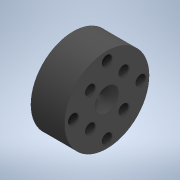
# Autodesk Inventor part: baseSoporte
Saved by Autodesk Inventor 2021.5 (Build 255421000, 421)
## iProperties
Created: 2024-11-19
Part Number: baseSoporte
Material: ABS NEGRO 4DLAB
Document SubType Name: Modeling
Designer: Joho_
Density: 0.894 g/cm^3
Appearance: Genérico(2)
Mass: 23.9494 g
Surface Area: 100.952 cm^2
Volume: 26.789 cm^3
Author: Joho_
## iProperties of the stored document _3DPrint.ipt
Created: 2024-11-25
Part Number: _3DPrint
Material: Genérico
Document SubType Name: Modeling
Designer: Joho_
Density: 1 g/cm^3
Appearance: Valor por defecto
Author: Joho_
Autodesk Inventor part; units mm, degrees
ref_plane "YZ Plane" through (0, 0, 0) normal (1, 0, 0) x (0, 1, 0)
sketch "Boceto2" plane through (0, 0, 0) normal (0, 0, 1) x (1, 0, 0)
  line L0 (0, 0) -> (-71.5, 0)
  line L1 (0, 10.9) -> (0, 0)
  line L2 (-68.2708, 0) -> (0, 0)
  line L3 (0, 10.9) -> (-68.1013, 9.2541)
  line L4 (-71.5, 0) -> (-56.9274, 0) construction
  line L5 (-71.5, 0) -> (-71.5, 8.5)
  line L6 (-71.5, 0) -> (-68, 0)
  arc A0 (-68, 9.2565) -> (-71.5, 8.5) centre (-67.8264, -0.0207) ccw
  line L7 (-68, 9.2565) -> (0, 10.9)
  line L8 (0, 0) -> (26.5, 0)
  line L9 (26.5, 0) -> (26.5, 7)
  line L10 (0, 0) -> (0, 9.9)
  line L11 (0, 0) -> (21, 0)
  line L12 (21, 0) -> (21, 9.5)
  line L13 (21, 9.5) -> (0, 9.9)
  line L14 (26.5, 0) -> (26.5, 8.5)
  arc A1 (26.5, 8.5) -> (21, 9.5) centre (21.692, -2.3188) ccw
  line L15 (26.5, 0) -> (29, 0)
  line L16 (29, 0) -> (29, 7)
  line L17 (29, 7) -> (26.5, 7)
  line L18 (29, 0) -> (29, 6.75)
  line L19 (29, 6.75) -> (31, 6.75)
  line L20 (31.8816, 0) -> (29, 0)
  line L21 (29, 0) -> (29, 6.75)
  line L22 (29, 6.75) -> (31, 6.75)
  line L23 (29, 0) -> (31, 0)
  ellipse E0 centre (31, 0) end of major axis (31, 6.75) minor radius 0.8816 (31.8816, 0) -> (31, 6.75) ccw
  line L24 (-71.5, 0) -> (-71.5, 7.25)
  line L25 (-71.5, 0) -> (-67, 0)
  line L26 (-71.5, 0) -> (-76, 0)
  line L27 (-76, 0) -> (-76, 6.75)
  line L28 (-76, 6.75) -> (-71.5, 7.25)
  line L29 (-76, 0) -> (-77, 0)
  line L30 (-77, 0) -> (-77, 6.5)
  line L31 (-77, 6.5) -> (-76, 6.75)
  line L32 (-77, 0) -> (-80.5, 0)
  line L33 (-80.5, 0) -> (-80.5, 4.15)
  line L34 (-80.5, 4.15) -> (-77, 6.5)
  line L35 (-80.5, 0) -> (-87.5, 0)
  line L36 (-87.5, 0) -> (-87.5, 4.15)
  line L37 (-87.5, 4.15) -> (-80.5, 4.15)
  line L38 (-80.5, 4.15) -> (-80.5, 0)
  line L39 (-87.5, 0) -> (-95, 0)
  line L40 (-95, 0) -> (-95, 0)
  line L41 (-92.25, 2.75) -> (-87.5, 2.75)
  line L42 (-87.5, 2.75) -> (-87.5, 0)
  arc A2 (-92.25, 2.75) -> (-95, 0) centre (-92.25, 0) ccw
  line L43 (-71.5, 8.5) -> (-71.5, 12.7399)
  arc A3 (-68.0867, 13.2556) -> (-71.5, 12.7399) centre (-67.8264, -0.0207) ccw
  line L44 (-68.0867, 13.2556) -> (-0.0966, 14.8988)
  line L45 (34.8792, 10.8985) -> (49.8792, 10.8985)
  line L46 (-71.5, 0) -> (-61.5, 0)
  line L47 (-61.5, 0) -> (-61.5, 13.4148)
  line L48 (-61.5, 14.4151) -> (-61.5, 20)
  line L49 (-61.5, 13.4148) -> (-61.5, 14.4151)
  line L50 (-61.5, 13.4148) -> (-58, 13.4148) construction
  circle A4 centre (-61.5, 13.4148) radius 1.5
  line L51 (-61.5, 13.4148) -> (-58.5, 13.4148)
  line L52 (-58.5, 13.4148) -> (-60, 10.8167)
  line L53 (-60, 10.8167) -> (-63, 10.8167)
  line L54 (-63, 10.8167) -> (-64.5, 13.4148)
  line L55 (-64.5, 13.4148) -> (-63, 16.0129)
  line L56 (-63, 16.0129) -> (-60, 16.0129)
  line L57 (-60, 16.0129) -> (-58.5, 13.4148)
  line L58 (-64.7321, 19.0129) -> (-67.9641, 13.4148)
  line L59 (-67.9641, 13.4148) -> (-64.7321, 7.8167)
  line L60 (-64.7321, 7.8167) -> (-58.2679, 7.8167)
  line L61 (-58.2679, 7.8167) -> (-55.0359, 13.4148)
  line L62 (-55.0359, 13.4148) -> (-58.2679, 19.0129)
  line L63 (-58.2679, 19.0129) -> (-64.7321, 19.0129)
  line L64 (-67.9641, 13.4148) -> (-55.0359, 13.4148)
  line L65 (49.8792, 0) -> (39.8792, 0)
  line L66 (-71.5, 0) -> (-10.8105, 0)
  line L67 (-10.8105, 0) -> (-10.8105, 14.6399)
  line L68 (-10.8105, 14.6399) -> (-10.8105, 27)
  circle A5 centre (-10.8105, 14.6399) radius 1.5
  line L69 (-10.8105, 14.6399) -> (-7.8105, 14.6399)
  line L70 (-10.8105, 14.6399) -> (-7.8105, 14.6399) construction
  line L71 (-7.8105, 14.6399) -> (-9.3105, 12.0418)
  line L72 (-9.3105, 12.0418) -> (-12.3105, 12.0418)
  line L73 (-12.3105, 12.0418) -> (-13.8105, 14.6399)
  line L74 (-13.8105, 14.6399) -> (-12.3105, 17.238)
  line L75 (-12.3105, 17.238) -> (-9.3105, 17.238)
  line L76 (-9.3105, 17.238) -> (-7.8105, 14.6399)
  line L77 (-14.0426, 20.238) -> (-17.2746, 14.6399)
  line L78 (-17.2746, 14.6399) -> (-14.0426, 9.0418)
  line L79 (-14.0426, 9.0418) -> (-7.5784, 9.0418)
  line L80 (-7.5784, 9.0418) -> (-4.3464, 14.6399)
  line L81 (-4.3464, 14.6399) -> (-7.5784, 20.238)
  line L82 (-7.5784, 20.238) -> (-14.0426, 20.238)
  line L83 (0, 10.9) -> (50, 10.9)
  line L84 (50, 10.9) -> (50, 14.9)
  line L85 (50, 14.9) -> (0, 14.9)
  line L86 (0, 14.9) -> (0, 10.9)
  line L87 (-0.0966, 14.8988) -> (0, 14.8988)
  line L88 (0, 0) -> (50, 0)
  line L89 (50, 0) -> (50, 10.9)
  line L90 (50, 10.9) -> (0, 10.9)
  line L91 (0, 10.9) -> (0, 0)
  point P0 (67.7333, -10.8479)
  point P1 (103.6012, -10.8479)
  point P2 (35.8517, 0)
  point P3 (7, 16)
  point P4 (-95, 2.75)
  dimension "d21" = 71.5
  dimension "d22" = 8.5
  dimension "d23" = 3.5
  dimension "d24" = 26.5
  dimension "d25" = 7
  dimension "d26" = 9.9
  dimension "d27" = 21
  dimension "d28" = 9.5
  dimension "d29" = 8.5
  dimension "d30" = 2.5
  dimension "d31" = 6.75
  dimension "d32" = 2
  dimension "d33" = 2
  dimension "d34" = 7.25
  dimension "d35" = 4.5
  dimension "d36" = 4.5
  dimension "d37" = 6.75
  dimension "d38" = 1
  dimension "d39" = 6.5
  dimension "d40" = 3.5
  dimension "d41" = 4.15
  dimension "d42" = 7
  dimension "d43" = 7.5
  dimension "d44" = 2.75
  dimension "d45" = 2.75
  dimension "d51" = 4
  dimension "d52" = 10
  dimension "d53" = 20
  dimension "d54" = 90
  dimension "d55" = 3
  dimension "d56" = 3
  dimension "d57" = 3
  dimension "d58" = 10
  dimension "d63" = 60.6895
  dimension "d64" = 3
  dimension "d65" = 3
  dimension "d66" = 0
  dimension "d67" = 3
  dimension "d89" = 50
  dimension "d90" = 4
  dimension "d91" = 121.5
  dimension "d92" = 50
  constraints: 184 end point, 19 horizontal, 17 point on line, 12 perpendicular, 10 coincident, 9 parallel, 9 point on circle, 6 centre point, 6 vertical, 2 collinear, 2 tangent, 40 other
  measures "d21" distance of L0.start L0.end
  measures "d22" distance of L0.end L5.end
  measures "d23" distance of L0.end L6.end
  measures "d24" distance of L0.start L8.end
  measures "d25" distance of L8.end L9.end
  measures "d26" distance of L0.start L10.end
  measures "d27" distance of L0.start L11.end
  measures "d28" distance of L11.end L12.end
  measures "d29" distance of L8.end L14.end
  measures "d30" distance of L8.end L15.end
  measures "d31" distance of L15.end L18.end
  measures "d32" distance of L18.end L19.end
  measures "d33" distance of L20.end L23.end
  measures "d34" distance of L0.end L24.end
  measures "d35" distance of L0.end L25.end
  measures "d36" distance of L0.end L26.end
  measures "d37" distance of L26.end L27.end
  measures "d38" distance of L26.end L29.end
  measures "d39" distance of L29.end L30.end
  measures "d40" distance of L29.end L32.end
  measures "d41" distance of L32.end L33.end
  measures "d42" distance of L36.end L37.end
  measures "d43" distance of point (-95, 2.75) L41.end
  measures "d44" distance of L39.end point (-95, 2.75)
  measures "d45" radius of A2
  measures "d51" radial gap between concentric circles of A0 A3
  measures "d52" distance of L0.end L46.end
  measures "d53" distance of L46.end L48.end
  measures "d54" angle of L47 L46
  measures "d55" diameter of A4
  measures "d56" distance of L51.start L51.end
  measures "d57" distance between parallel lines of L55 L58
  measures "d58" distance of L65.start L65.end
  measures "d63" distance of L0.end L66.end
  measures "d64" diameter of A5
  measures "d65" distance of L69.start L69.end
  measures "d66" distance between parallel lines of L69 L70
  measures "d67" distance between parallel lines of L74 L77
  measures "d89" distance of L85.end L84.end
  measures "d90" distance of L84.end L83.end
  measures "d91" distance between parallel lines of L84 L24
  measures "d92" distance between parallel lines of L86 L84
sketch "Boceto4" plane through (0, 0, 0) normal (1, 0, 0) x (0, 1, 0)
  line L0 (0, 0) -> (0, 20)
  circle A0 centre (20, 0) radius 3
  circle A1 centre (0, 20) radius 3
  circle A2 centre (-20, 0) radius 3
  circle A3 centre (0, 0) radius 12.5
  circle A4 centre (0, 0) radius 20
  circle A5 centre (0, 0) radius 20
  circle A6 centre (0, 0) radius 20
  circle A7 centre (0, 0) radius 25
  circle A8 centre (0, 0) radius 20
  circle A9 centre (0, -20) radius 3
  line L1 (0, -20) -> (3.5355, -16.4645) construction
  circle A10 centre (9.9038, -9.9038) radius 1.5
  line L2 (0, 0) -> (6.2936, 0)
  line L3 (15, 15) -> (-15, 15)
  line L4 (-15, 15) -> (-15, -15)
  line L5 (-15, -15) -> (15, -15)
  line L6 (15, -15) -> (15, 15)
  line L7 (15, 15) -> (-15, -15) construction
  line L8 (8.3161, -12.6538) -> (6.7284, -9.9038)
  line L9 (6.7284, -9.9038) -> (8.3161, -7.1538)
  line L10 (8.3161, -7.1538) -> (11.4915, -7.1538)
  line L11 (11.4915, -7.1538) -> (13.0792, -9.9038)
  line L12 (13.0792, -9.9038) -> (11.4915, -12.6538)
  line L13 (11.4915, -12.6538) -> (8.3161, -12.6538)
  circle A11 centre (9.9038, 9.9038) radius 1.5
  line L14 (8.3161, 12.6538) -> (6.7284, 9.9038)
  line L15 (6.7284, 9.9038) -> (8.3161, 7.1538)
  line L16 (8.3161, 7.1538) -> (11.4915, 7.1538)
  line L17 (11.4915, 7.1538) -> (13.0792, 9.9038)
  line L18 (13.0792, 9.9038) -> (11.4915, 12.6538)
  line L19 (11.4915, 12.6538) -> (8.3161, 12.6538)
  circle A12 centre (-9.9038, -9.9038) radius 1.5
  line L20 (-8.3161, -12.6538) -> (-6.7284, -9.9038)
  line L21 (-6.7284, -9.9038) -> (-8.3161, -7.1538)
  line L22 (-8.3161, -7.1538) -> (-11.4915, -7.1538)
  line L23 (-11.4915, -7.1538) -> (-13.0792, -9.9038)
  line L24 (-13.0792, -9.9038) -> (-11.4915, -12.6538)
  line L25 (-11.4915, -12.6538) -> (-8.3161, -12.6538)
  line L26 (-13.0792, 9.9038) -> (-11.4915, 12.6538)
  line L27 (-8.3161, 7.1538) -> (-11.4915, 7.1538)
  line L28 (-6.7284, 9.9038) -> (-8.3161, 7.1538)
  line L29 (-11.4915, 7.1538) -> (-13.0792, 9.9038)
  circle A13 centre (-9.9038, 9.9038) radius 1.5
  line L30 (-8.3161, 12.6538) -> (-6.7284, 9.9038)
  line L31 (-11.4915, 12.6538) -> (-8.3161, 12.6538)
  circle A14 centre (9.9038, 9.9038) radius 3
  circle A15 centre (9.9038, -9.9038) radius 3
  circle A16 centre (-9.9038, 9.9038) radius 3
  circle A17 centre (-9.9038, -9.9038) radius 3
  point P0 (20, 0)
  point P1 (-6.2936, 0)
  dimension "d105" = 40
  dimension "d104" = 50
  dimension "d107" = 6
  dimension "d108" = 360
  dimension "d110" = 25
  dimension "d126" = 3
  dimension "d132" = 30
  dimension "d133" = 30
  dimension "d270" = 6
  dimension "d271" = 6
  dimension "d272" = 6
  dimension "d273" = 6
  constraints: 64 end point, 25 symmetric about line, 14 centre point, 12 coincident, 2 horizontal, 2 horizontal alignment, 2 parallel, 2 vertical alignment, 1 midpoint, 1 perpendicular, 43 other
  measures "d104" diameter of A7
  measures "d107" diameter of A1
  measures "d110" diameter of A3
  measures "d126" diameter of A10
  measures "d132" distance of L5.end L4.end
  measures "d133" distance of L4.end L3.end
  measures "d270" diameter of A14
  measures "d271" diameter of A15
  measures "d272" diameter of A16
  measures "d273" diameter of A17
sketch "Boceto3" plane through (0, 0, 0) normal (1, 0, 0) x (0, 1, 0)
  line L0 (0, 0) -> (20, 0) construction
  line L1 (0, 0) -> (14.1421, 14.1421)
  circle A0 centre (0, 20) radius 3
  circle A1 centre (14.1421, -14.1421) radius 3
  circle A2 centre (14.1421, 14.1421) radius 3
  circle A3 centre (-14.1421, 14.1421) radius 3
  circle A4 centre (0, 0) radius 12.5
  circle A5 centre (0, 0) radius 20
  circle A6 centre (0, 0) radius 20
  circle A7 centre (0, 0) radius 20
  circle A8 centre (0, 0) radius 25
  circle A9 centre (0, 0) radius 20
  circle A10 centre (-14.1421, -14.1421) radius 3
  line L2 (20, 0) -> (20, 4)
  line L3 (20, 4) -> (23.4641, 2)
  line L4 (23.4641, 2) -> (23.4641, -2)
  line L5 (23.4641, -2) -> (20, -4)
  line L6 (20, -4) -> (16.5359, -2)
  line L7 (16.5359, -2) -> (16.5359, 2)
  line L8 (16.5359, 2) -> (20, 4)
  line L9 (-4, 20) -> (-2, 23.4641)
  line L10 (-2, 23.4641) -> (2, 23.4641)
  line L11 (2, 23.4641) -> (4, 20)
  line L12 (4, 20) -> (2, 16.5359)
  line L13 (-2, 16.5359) -> (-4, 20)
  line L14 (2, 16.5359) -> (-2, 16.5359)
  line L15 (-20, -4) -> (-23.4641, -2)
  line L16 (-23.4641, -2) -> (-23.4641, 2)
  line L17 (-23.4641, 2) -> (-20, 4)
  line L18 (-20, 4) -> (-16.5359, 2)
  line L19 (-16.5359, -2) -> (-20, -4)
  line L20 (-16.5359, 2) -> (-16.5359, -2)
  line L21 (4, -20) -> (2, -23.4641)
  line L22 (2, -23.4641) -> (-2, -23.4641)
  line L23 (-2, -23.4641) -> (-4, -20)
  line L24 (-4, -20) -> (-2, -16.5359)
  line L25 (2, -16.5359) -> (4, -20)
  line L26 (-2, -16.5359) -> (2, -16.5359)
  circle A11 centre (20, 0) radius 2
  circle A12 centre (0, 20) radius 2
  circle A13 centre (-20, 0) radius 2
  circle A14 centre (0, -20) radius 2
  line L27 (-14.1421, -14.1421) -> (-17.6777, -17.6777)
  line L28 (-14.1421, -14.1421) -> (-9.1421, -14.1421) construction
  line L29 (-17.6777, -17.6777) -> (17.6777, -17.6777)
  line L30 (17.6777, -17.6777) -> (17.6777, 17.6777)
  line L31 (17.6777, -17.6777) -> (59.3553, -17.6777) construction
  line L32 (17.6777, 17.6777) -> (-17.6777, 17.6777)
  line L33 (17.6777, 17.6777) -> (68.3553, 17.6777) construction
  line L34 (-17.6777, 17.6777) -> (-17.6777, -17.6777)
  dimension "d75" = 40
  dimension "d74" = 50
  dimension "d76" = 45
  dimension "d77" = 6
  dimension "d78" = 360
  dimension "d79" = 6
  dimension "d80" = 25
  dimension "d81" = 4
  dimension "d82" = 360
  dimension "d83" = 4
  dimension "d84" = 360
  dimension "d85" = 135
  dimension "d86" = 45
  dimension "d87" = 90
  dimension "d88" = 180
  constraints: 70 end point, 12 centre point, 11 coincident, 6 point on circle, 4 horizontal, 2 coincident with centre, 2 equal length, 2 vertical, 97 other
  measures "d74" diameter of A8
  measures "d76" angle of L0 L1
  measures "d77" diameter of A2
  measures "d79" diameter of A0
  measures "d80" diameter of A4
  measures "d81" distance of L0.end L2.end
  measures "d83" diameter of A11
  measures "d85" angle of L27 L28
  measures "d86" angle of L29 L27
  measures "d87" angle of L31 L30
  measures "d88" angle of L32 L33
extrude "Extrusión2" add sketch "Boceto4" along normal blind 50 and the other way blind 71.5 contours L3 A4 L6 L5 L4 | A3 A14 L14 L15 L16 A15 L10 L9 L8 A17 L20 L21 L22 A16 L27 L28 L30 | A14 L14 A3 | A3 L14 A14 | A16 L30 A3 | A3 L30 A16 | L3 L6 A4 | A4 L4 L3 | L14 A14 L19 L18 L17 L16 A3 | A3 L16 A14 L15 L14 | L14 L19 A14 | A14 L15 L14 | L30 A16 L28 L27 A3 | A3 L27 A16 L29 L26 L31 L30 | L30 L28 A16 | A16 L31 L30 | L16 A14 A3 | A3 A14 L16 | A14 L19 | L15 A14 | L27 A16 A3 | A3 A16 L27 | L31 A16 | L6 L5 A4 | A4 L5 L4 | L16 L15 A14 | A14 L17 L16 | L19 L18 A14 | A16 L28 L27 | L27 L29 A16 | A16 L28 | A16 L26 L31 | L17 A14 | A14 L18 | A17 L22 A3 | A3 L22 A17 | A16 L29 | L26 A16 | A15 L10 A3 | A3 L10 A15 | A14 L18 L17 | L22 A17 L21 L20 A3 | A3 L20 A17 L25 L24 L23 L22 | L22 L21 A17 | A17 L23 L22 | L29 L26 A16 | L10 A15 L11 L12 L13 L8 A3 | A3 L8 A15 L9 L10 | L10 L11 A15 | A15 L9 L10 | L20 A17 A3 | A3 A17 L20 | A17 L21 | L23 A17 | L8 A15 A3 | A3 A15 L8 | A15 L11 | L9 A15 | L20 L25 A17 | A17 L21 L20 | A17 L24 L23 | A15 L13 L8 | L8 L9 A15 | L11 L12 A15 | A17 L25 | L24 A17 | L13 A15 | L25 L24 A17 | A15 L12 L13 | A15 L12 | A10 | A11 | A12 | A13
revolve "Revolución2" cut sketch "Boceto2" angle 360 about axis through (-71.5, 0, 0) along (1, 0, 0) contours L0 L67 L79 L80 L3 L1 | L1 L13 L12 L8 | L0 L47 L60 L61 L3 L78 L79 L67 | L1 L83 L45 L89 L88 L65 E0 L19 L16 L17 L14 A1 L13 | L12 A1 L14 L9 L8 | L0 L5 A0 L3 L59 L60 L47 | L79 L78 L3 L67 | L67 L3 L80 L79 | L9 L17 L16 L15 | L60 L59 L3 L47 | L47 L3 L61 L60 | L16 L19 E0 L20
sketch "Boceto5" plane through (50, 0, 0) normal (1, 0, 0) x (0, 0, -1)
  line L0 (0, 0) -> (0, 20)
  circle A0 centre (20, 0) radius 3
  circle A1 centre (0, 20) radius 3
  circle A2 centre (-20, 0) radius 3
  circle A3 centre (0, 0) radius 20
  circle A4 centre (0, 0) radius 20
  circle A5 centre (0, 0) radius 20
  circle A6 centre (0, 0) radius 20
  circle A7 centre (0, -20) radius 3
  line L1 (0, -20) -> (3.5355, -16.4645) construction
  circle A8 centre (9.9038, -9.9038) radius 1.5
  line L2 (0, 0) -> (6.2936, 0)
  line L3 (15, 15) -> (-15, 15)
  line L4 (-15, 15) -> (-15, -15)
  line L5 (-15, -15) -> (15, -15)
  line L6 (15, -15) -> (15, 15)
  line L7 (15, 15) -> (-15, -15) construction
  line L8 (8.3161, -12.6538) -> (6.7284, -9.9038)
  line L9 (6.7284, -9.9038) -> (8.3161, -7.1538)
  line L10 (8.3161, -7.1538) -> (11.4915, -7.1538)
  line L11 (11.4915, -7.1538) -> (13.0792, -9.9038)
  line L12 (13.0792, -9.9038) -> (11.4915, -12.6538)
  line L13 (11.4915, -12.6538) -> (8.3161, -12.6538)
  line L14 (13.0792, 9.9038) -> (11.4915, 12.6538)
  line L15 (8.3161, 7.1538) -> (11.4915, 7.1538)
  line L16 (6.7284, 9.9038) -> (8.3161, 7.1538)
  line L17 (11.4915, 7.1538) -> (13.0792, 9.9038)
  circle A9 centre (9.9038, 9.9038) radius 1.5
  line L18 (8.3161, 12.6538) -> (6.7284, 9.9038)
  line L19 (11.4915, 12.6538) -> (8.3161, 12.6538)
  line L20 (-8.3161, -7.1538) -> (-11.4915, -7.1538)
  line L21 (-13.0792, -9.9038) -> (-11.4915, -12.6538)
  line L22 (-8.3161, -12.6538) -> (-6.7284, -9.9038)
  circle A10 centre (-9.9038, -9.9038) radius 1.5
  line L23 (-6.7284, -9.9038) -> (-8.3161, -7.1538)
  line L24 (-6.7284, 9.9038) -> (-8.3161, 7.1538)
  line L25 (-8.3161, 7.1538) -> (-11.4915, 7.1538)
  line L26 (-11.4915, 7.1538) -> (-13.0792, 9.9038)
  line L27 (-13.0792, 9.9038) -> (-11.4915, 12.6538)
  line L28 (-8.3161, 12.6538) -> (-6.7284, 9.9038)
  line L29 (-11.4915, 12.6538) -> (-8.3161, 12.6538)
  line L30 (-11.4915, -7.1538) -> (-13.0792, -9.9038)
  circle A11 centre (-9.9038, 9.9038) radius 1.5
  line L31 (-11.4915, -12.6538) -> (-8.3161, -12.6538)
  circle A12 centre (0, 0) radius 25
  point P0 (20, 0)
  point P1 (-6.2936, 0)
  dimension "d144" = 40
  dimension "d145" = 6
  dimension "d146" = 360
  dimension "d148" = 3
  dimension "d149" = 30
  dimension "d150" = 30
  dimension "d182" = 50
  constraints: 64 end point, 25 symmetric about line, 9 centre point, 7 coincident, 2 horizontal, 2 horizontal alignment, 2 parallel, 2 vertical alignment, 1 midpoint, 1 perpendicular, 43 other
  measures "d145" diameter of A1
  measures "d148" diameter of A8
  measures "d149" distance of L5.end L4.end
  measures "d150" distance of L4.end L3.end
  measures "d182" diameter of A12
extrude "Extrusión3" cut sketch "Boceto5" against normal blind 20 contours A8 | A9 | A10 | A11
ref_plane "Plano de trabajo1" through (45, 0, 0) normal (1, 0, 0) x (0, 0, -1)
sketch "Boceto8" plane through (45, 0, 0) normal (1, 0, 0) x (0, 0, -1)
  line L0 (0, 0) -> (0, 20)
  circle A0 centre (20, 0) radius 3
  circle A1 centre (0, 20) radius 3
  circle A2 centre (-20, 0) radius 3
  circle A3 centre (0, 0) radius 20
  circle A4 centre (0, 0) radius 20
  circle A5 centre (0, 0) radius 20
  circle A6 centre (0, 0) radius 20
  circle A7 centre (0, -20) radius 3
  line L1 (0, -20) -> (3.5355, -16.4645) construction
  circle A8 centre (9.9038, -9.9038) radius 1.5
  line L2 (0, 0) -> (6.2936, 0)
  line L3 (15, 15) -> (-15, 15)
  line L4 (-15, 15) -> (-15, -15)
  line L5 (-15, -15) -> (15, -15)
  line L6 (15, -15) -> (15, 15)
  line L7 (8.3161, -12.6538) -> (6.7284, -9.9038)
  line L8 (6.7284, -9.9038) -> (8.3161, -7.1538)
  line L9 (8.3161, -7.1538) -> (11.4915, -7.1538)
  line L10 (11.4915, -7.1538) -> (13.0792, -9.9038)
  line L11 (13.0792, -9.9038) -> (11.4915, -12.6538)
  line L12 (11.4915, -12.6538) -> (8.3161, -12.6538)
  line L13 (13.0792, 9.9038) -> (11.4915, 12.6538)
  line L14 (8.3161, 7.1538) -> (11.4915, 7.1538)
  line L15 (6.7284, 9.9038) -> (8.3161, 7.1538)
  line L16 (11.4915, 7.1538) -> (13.0792, 9.9038)
  circle A9 centre (9.9038, 9.9038) radius 1.5
  line L17 (8.3161, 12.6538) -> (6.7284, 9.9038)
  line L18 (11.4915, 12.6538) -> (8.3161, 12.6538)
  line L19 (-8.3161, -7.1538) -> (-11.4915, -7.1538)
  line L20 (-13.0792, -9.9038) -> (-11.4915, -12.6538)
  line L21 (-8.3161, -12.6538) -> (-6.7284, -9.9038)
  circle A10 centre (-9.9038, -9.9038) radius 1.5
  line L22 (-6.7284, -9.9038) -> (-8.3161, -7.1538)
  line L23 (-6.7284, 9.9038) -> (-8.3161, 7.1538)
  line L24 (-8.3161, 7.1538) -> (-11.4915, 7.1538)
  line L25 (-11.4915, 7.1538) -> (-13.0792, 9.9038)
  line L26 (-13.0792, 9.9038) -> (-11.4915, 12.6538)
  line L27 (-8.3161, 12.6538) -> (-6.7284, 9.9038)
  line L28 (-11.4915, 12.6538) -> (-8.3161, 12.6538)
  line L29 (-11.4915, -7.1538) -> (-13.0792, -9.9038)
  circle A11 centre (-9.9038, 9.9038) radius 1.5
  line L30 (-11.4915, -12.6538) -> (-8.3161, -12.6538)
  line L31 (15, -15) -> (15, 15)
  line L32 (11.4915, -12.6538) -> (15, -12.6538)
  line L33 (15, -12.6538) -> (15, -7.1538)
  line L34 (15, -7.1538) -> (11.4915, -7.1538)
  line L35 (11.4915, -7.1538) -> (11.4915, -12.6538)
  line L36 (11.4915, 7.1538) -> (15, 7.1538)
  line L37 (15, 7.1538) -> (15, 12.6538)
  line L38 (15, 12.6538) -> (11.4915, 12.6538)
  line L39 (11.4915, 12.6538) -> (11.4915, 7.1538)
  line L40 (-11.4915, 12.6538) -> (-17.8424, 12.6538)
  line L41 (-17.8424, 12.6538) -> (-17.8424, 7.1538)
  line L42 (-17.8424, 7.1538) -> (-11.4915, 7.1538)
  line L43 (-11.4915, 7.1538) -> (-11.4915, 12.6538)
  line L44 (-11.4915, -7.1538) -> (-17.8424, -7.1538)
  line L45 (-17.8424, -7.1538) -> (-17.8424, -12.6538)
  line L46 (-17.8424, -12.6538) -> (-11.4915, -12.6538)
  line L47 (-11.4915, -12.6538) -> (-11.4915, -7.1538)
  point P0 (20, 0)
  point P1 (-6.2936, 0)
  dimension "d172" = 40
  dimension "d173" = 6
  dimension "d174" = 360
  dimension "d175" = 3
  dimension "d176" = 30
  dimension "d177" = 30
  dimension "d178" = 5.5
  dimension "d179" = 5.5
  constraints: 96 end point, 8 centre point, 6 coincident, 4 parallel, 2 horizontal, 2 horizontal alignment, 2 perpendicular, 2 point on line, 2 vertical alignment, 40 other
  measures "d173" diameter of A1
  measures "d175" diameter of A8
  measures "d176" distance of L6.start L4.end
  measures "d177" distance of L4.end L3.end
  measures "d178" distance of L33.end L32.end
  measures "d179" distance of L37.end L36.end
extrude "Extrusión4" cut sketch "Boceto8" along normal mid plane 2.5 contours L6 L36 L16 L13 L38 | L40 L4 L42 L41 A3 | A3 L41 L40 | L40 L26 L25 L42 L4 | L39 L14 L15 L17 L18 | L13 L16 L39 | L43 L25 L26 | L28 L27 L23 L24 L43 | L6 L32 L11 L10 L34 | L44 L29 L20 L46 L4 | L4 L46 A3 L45 L44 | L35 L12 L7 L8 L9 | L10 L11 L35 | L47 L20 L29 | L19 L22 L21 L30 L47 | A3 L46 L45 | A8 | A9 | A10 | A11
sketch "Boceto9" plane through (50, 0, 0) normal (1, 0, 0) x (0, 0, -1)
  circle A0 centre (20, 0) radius 3
  circle A1 centre (0, 20) radius 3
  circle A2 centre (-20, 0) radius 3
  circle A3 centre (0, 0) radius 12.5
  circle A4 centre (0, 0) radius 20
  circle A5 centre (0, 0) radius 20
  circle A6 centre (0, 0) radius 20
  circle A7 centre (0, 0) radius 25
  circle A8 centre (0, 0) radius 20
  circle A9 centre (0, -20) radius 3
  line L0 (0, -20) -> (3.5355, -16.4645) construction
  line L1 (0, 0) -> (6.2936, 0)
  circle A10 centre (0, 0) radius 2
  circle A11 centre (0, 0) radius 4
  line L2 (-15, 15) -> (15, 15)
  line L3 (15, 15) -> (15, -15)
  line L4 (15, -15) -> (-15, -15)
  line L5 (-15, -15) -> (-15, 15)
  line L6 (-15, 15) -> (15, -15) construction
  line L7 (15, 15) -> (-15, -15) construction
  point P0 (20, 0)
  point P1 (-6.2936, 0)
  point P2 (-15, -13.2288)
  point P3 (-19.775, -2.9916)
  point P4 (-19.775, 2.9916)
  point P5 (-15, 13.2288)
  point P6 (-13.2288, 15)
  point P7 (-2.9916, 19.775)
  point P8 (2.9916, 19.775)
  point P9 (13.2288, 15)
  dimension "d187" = 40
  dimension "d186" = 50
  dimension "d188" = 6
  dimension "d189" = 360
  dimension "d190" = 25
  dimension "d194" = 4
  dimension "d195" = 8
  dimension "d244" = 30
  dimension "d245" = 30
  constraints: 16 end point, 10 coincident, 8 centre point, 2 horizontal, 2 horizontal alignment, 2 midpoint, 2 parallel, 1 perpendicular, 1 vertical alignment, 28 other
  measures "d186" diameter of A7
  measures "d188" diameter of A1
  measures "d190" diameter of A3
  measures "d194" diameter of A10
  measures "d195" diameter of A11
  measures "d244" distance of L3.end L4.end
  measures "d245" distance of L2.end L3.end
extrude "Extrusión5" add sketch "Boceto9" along normal blind 10 contours A0 A4 L3 | L3 A4 L4 L5 L2 | A4 L2 L3 | L3 L4 A4 | L2 A4 A1 | A4 A9 L4 | A4 L5 L2 | L4 L5 A4 | L5 A4 A2 | A3 | A7 | A11
ref_plane "Plano de trabajo2" through (0, 0, 15) normal (0, 0, 1) x (1, 0, 0)
extrude "Extrusión10" add sketch "Boceto9" against normal blind 10 contours A0 A4 L3 | L2 A4 A1 | A4 A9 L4 | L5 A4 A2 | A7
chamfer "Chaflán1" distance 1 angle 45 4 edges at (40, 0, -17) (40, 20.225, 2.9916) (40, -2.9916, 20.225) (40, -20, 3)
chamfer "Chaflán2" distance 5 angle 45 1 edges at (60, 0, 2)
sketch "Boceto12" plane through (-71.5, 0, 0) normal (-1, 0, 0) x (0, 0, 1)
  line L0 (15, -15) -> (-15, -15)
  line L1 (-15, -15) -> (-15, 15)
  line L2 (-15, 15) -> (15, 15)
  line L3 (15, 15) -> (15, -15)
  line L4 (15, -15) -> (-15, 15) construction
  line L5 (-15, -15) -> (15, 15) construction
  point P0 (0, 0)
  dimension "d261" = 30
  dimension "d262" = 30
  constraints: 12 end point, 2 midpoint, 2 parallel, 1 horizontal, 1 perpendicular
  measures "d261" distance of L1.end L2.end
  measures "d262" distance of L0.end L1.end
extrude "Extrusión12" cut sketch "Boceto12" against normal blind 121.5
extrude "Extrusión13" cut sketch "Boceto4" along normal blind 100 contours A10 | A11 | A12 | A13
sketch "Boceto13" plane through (60, 0, 0) normal (1, 0, 0) x (0, 0, -1)
  circle A0 centre (-9.9038, -9.9038) radius 2.5
  circle A1 centre (-9.9038, 9.9038) radius 2.5
  circle A2 centre (-20, 0) radius 3
  circle A3 centre (0, 20) radius 3
  circle A4 centre (20, 0) radius 3
  circle A5 centre (0, -20) radius 3
  circle A6 centre (0, 0) radius 25
  circle A7 centre (0, 0) radius 7
  circle A8 centre (9.9038, 9.9038) radius 2.5
  circle A9 centre (9.9038, -9.9038) radius 2.5
  circle A10 centre (-9.9038, 9.9038) radius 3
  circle A11 centre (-9.9038, -9.9038) radius 3
  circle A12 centre (9.9038, -9.9038) radius 3
  circle A13 centre (9.9038, 9.9038) radius 3
  dimension "d274" = 6
  dimension "d277" = 360
  constraints: 23 centre point, 1 coincident, 9 other
  measures "d274" diameter of A10
extrude "Extrusión14" cut sketch "Boceto13" against normal blind 5 contours A0 | A1 | A8 | A9 | A10 | A11 | A12 | A13
chamfer "Chaflán4" distance 1.5 angle 45 4 edges at (55, 8.4038, 9.9038) (55, 8.4038, -9.9038) (55, -11.4038, 9.9038) (55, -11.4038, -9.9038)
